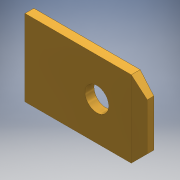
# Autodesk Inventor part: Toggle_Pin_Copper
Saved by Autodesk Inventor 2016 (Build 200138000, 138)
## iProperties
Created: 2016-04-13
Part Number: Toggle_Pin_Copper
Material: Brass, Soft Yellow
Document SubType Name: Modeling
Designer: agmle
Density: 8.47 g/cm^3
Appearance: Brass - Satin
Author: agmle
Autodesk Inventor part; units mm, degrees
ref_plane "YZ Plane" through (0, 0, 0) normal (1, 0, 0) x (0, 1, 0)
ref_plane "XZ Plane" through (0, 0, 0) normal (0, 1, 0) x (-1, 0, 0)
ref_plane "XY Plane" through (0, 0, 0) normal (0, 0, 1) x (1, 0, 0)
sketch "Sketch1" plane through (0, 0, 0) normal (0, 1, 0) x (-1, 0, 0)
  line L0 (5.105, 3.225) -> (-3.855, 3.225)
  line L1 (-5.105, 1.975) -> (-5.105, -1.975)
  line L2 (-3.855, -3.225) -> (5.105, -3.225)
  line L3 (5.105, -3.225) -> (5.105, 3.225)
  line L4 (5.105, 0) -> (-5.105, 0) construction
  line L5 (-3.855, 3.225) -> (-5.105, 1.975)
  line L6 (-5.105, -1.975) -> (-3.855, -3.225)
  line L7 (-4.48, 2.6) -> (-1.88, 0) construction
  line L8 (-4.48, -2.6) -> (-1.88, 0) construction
  circle A0 centre (-0.955, 0) radius 1
  point P0 (0, 0)
  point P1 (0, 0)
  dimension "d0" = 6.45
  dimension "d1" = 10.21
  dimension "d2" = 1.25
  dimension "d3" = 2
  dimension "d4" = 3.15
  constraints: 18 end point, 6 perpendicular, 5 midpoint, 2 parallel, 2 point on line, 1 centre point, 1 coincident, 1 horizontal
  measures "d0" distance between parallel lines of L2 L0
  measures "d1" distance between parallel lines of L1 L3
  measures "d2" distance from line of L0.end L1
  measures "d3" diameter of A0
  measures "d4" distance edge to line of A0 L1
extrude "Extrusion1" add sketch "Sketch1" along normal blind 0.75
chamfer "Chamfer1" distance 1.25 distance2 0.1 1 edges at (5.105, 0.75, 0) measured on face at (4.605, 0.75, 0)
chamfer "Chamfer2" distance 0.1 distance2 1.25 1 edges at (5.105, 0, 0) measured on face at (5.105, 0.5, 0)
body "Solid1"
